BoitierD1Relais (Autodesk Fusion 360 design; units mm, degrees)
Autodesk Fusion 360 part; units mm, degrees
sketch "Esquisse1" plane through (0, 0, 0) normal (0, 0, 1) x (1, 0, 0) in component "Boitier"
  line L0 (-18, 13.5) -> (18, 13.5)
  line L1 (18, 13.5) -> (18, -13.5)
  line L2 (18, -13.5) -> (-18, -13.5)
  line L3 (-18, -13.5) -> (-18, 13.5)
  line L4 (-18, 13.5) -> (18, -13.5) construction
  line L5 (18, 13.5) -> (-18, -13.5) construction
  line L6 (19.5, -15) -> (-19.5, -15)
  line L7 (-19.5, -15) -> (-19.5, 15)
  line L8 (-19.5, 15) -> (19.5, 15)
  line L9 (19.5, 15) -> (19.5, -15)
  dimension "d4" = 36
  dimension "d5" = 27
  constraint horizontal L0
  constraint perpendicular L0 L1
  constraint parallel L0 L2
  constraint parallel L1 L3
  constraint coincident L4 origin
  constraint coincident L5 origin
  measures "d4" distance of L1.end L2.end
  measures "d5" distance of L0.end L1.end
extrude "Extrusion1" add sketch "Esquisse1" along normal blind 1.5 contours L0 L1 L2 L3 makes body 1 in component "Boitier"
extrude "Extrusion2" add sketch "Esquisse1" along normal blind 33 bodies 1 in component "Boitier"
fillet "Congé1" radius 3 3 edges at (19.5, -15, 16.5) (19.5, 15, 16.5) (-19.5, 15, 16.5) on bodies 1 in component "Boitier"
fillet "Congé2" radius 3 1 edges at (-19.5, -15, 16.5) on bodies 1 in component "Boitier"
fillet "Congé3" radius 1.5 1 edges at (18, 13.5, 17.25) on bodies 1 in component "Boitier"
fillet "Congé4" radius 1.5 1 edges at (18, -13.5, 17.25) on bodies 1 in component "Boitier"
fillet "Congé5" radius 1.5 1 edges at (-18, -13.5, 17.25) on bodies 1 in component "Boitier"
fillet "Congé6" radius 1.5 1 edges at (-18, 13.5, 17.25) on bodies 1 in component "Boitier"
fillet "Congé7" radius 0.1 8 edges at (-18.6213, -14.1213, 33) (0, -15, 33) (18.6213, -14.1213, 33) (19.5, 0, 33) (18.6213, 14.1213, 33) (0, 15, 33) (-18.6213, 14.1213, 33) (-19.5, 0, 33) on bodies 1 in component "Boitier"
sketch "Esquisse3" plane through (19.5, 0, 0) normal (1, 0, 0) x (0, 1, 0) in component "Boitier"
  line L0 (-12, 0) -> (12, 0)
  line L1 (6.5, 7.5) -> (-6.5, 7.5)
  line L2 (-6.5, 7.5) -> (-6.5, 1.5)
  line L3 (-6.5, 1.5) -> (6.5, 1.5)
  line L4 (6.5, 1.5) -> (6.5, 7.5)
  line L5 (6.5, 7.5) -> (-6.5, 1.5) construction
  line L6 (-6.5, 7.5) -> (6.5, 1.5) construction
  line L7 (15, 0) -> (-15, 0)
  line L8 (12, 32.9) -> (-12, 32.9)
  line L9 (-12, 32.9) -> (-12, 0)
  line L10 (12, 0) -> (12, 32.9)
  point P0 (0, 4.5)
  dimension "d31" = 13
  dimension "d32" = 6
  dimension "d34" = 1.5
  constraint horizontal L1
  constraint perpendicular L1 L2
  constraint parallel L1 L3
  constraint parallel L2 L4
  constraint coincident L5 P0
  constraint coincident L6 P0
  measures "d31" distance of L2.end L3.end
  measures "d32" distance of L1.end L2.end
  measures "d34" distance of L3 L7
extrude "Extrusion3" cut sketch "Esquisse3" against normal blind 1.7 contours L1 L2 L3 L4 bodies 1 in component "Boitier"
sketch "Esquisse4" plane through (-19.5, 0, 0) normal (-1, 0, 0) x (0, -1, 0) in component "Boitier"
  line L0 (-12, 0) -> (12, 0)
  circle A0 centre (0, 4.95) radius 2
  line L1 (12, 32.9) -> (-12, 32.9)
  line L2 (-12, 32.9) -> (-12, 0)
  line L3 (12, 0) -> (12, 32.9)
  dimension "d38" = 4
  dimension "d39" = 4.95
  measures "d38" diameter of A0
  measures "d39" distance of origin A0.centre
extrude "Extrusion4" cut sketch "Esquisse4" against normal blind 1.7 contours A0 bodies 1 in component "Boitier"
sketch "Esquisse1 (2)" plane through (0, 0, 0) normal (0, 0, 1) x (1, 0, 0) in component "Couvercle"
  line L0 (96, 38.5) -> (57, 38.5)
  line L1 (57, 38.5) -> (57, 8.5)
  line L2 (57, 8.5) -> (96, 8.5)
  line L3 (96, 8.5) -> (96, 38.5)
  line L4 (96, 38.5) -> (57, 8.5) construction
  line L5 (57, 38.5) -> (96, 8.5) construction
  point P0 (76.5, 23.5)
  dimension "d77" = 39
  dimension "d78" = 30
  constraint horizontal L0
  constraint perpendicular L0 L1
  constraint parallel L0 L2
  constraint parallel L1 L3
  constraint coincident L4 P0
  constraint coincident L5 P0
  measures "d77" distance of L1.end L2.end
  measures "d78" distance of L0.end L1.end
extrude "Extrusion1'" add sketch "Esquisse1 (2)" along normal blind 1.5 separate body makes body 2 in component "Couvercle"
sketch "Esquisse2" plane through (0, 0, 1.5) normal (0, 0, 1) x (-1, 0, 0) in component "Couvercle"
  line L0 (-96, -8.5) -> (-96, -38.5)
  line L1 (-96, -38.5) -> (-57, -38.5)
  line L2 (-57, -38.5) -> (-57, -8.5)
  line L3 (-57, -8.5) -> (-96, -8.5)
  line L4 (-58.55, -36.95) -> (-94.45, -36.95)
  line L5 (-94.45, -36.95) -> (-94.45, -10.05)
  line L6 (-94.45, -10.05) -> (-58.55, -10.05)
  line L7 (-58.55, -10.05) -> (-58.55, -36.95)
  dimension "d81" = 35.9
  dimension "d82" = 26.9
  dimension "d83" = 1.55
  dimension "d84" = 1.55
  constraint horizontal L4
  constraint vertical L5
  constraint horizontal L6
  constraint vertical L7
  measures "d81" distance of L4.start L4.end
  measures "d82" distance of L4.start L6.end
  measures "d83" distance of L2 L7
  measures "d84" distance of L1 L4
extrude "Extrusion2'" add sketch "Esquisse2" along normal blind 2.25 contours L4 L5 L6 L7 bodies 2 in component "Couvercle"
sketch "Esquisse3 (2)" plane through (0, 0, 3.75) normal (0, 0, 1) x (-1, 0, 0) in component "Couvercle"
  line L0 (-58.55, -10.05) -> (-94.45, -10.05)
  line L1 (-94.45, -10.05) -> (-94.45, -36.95)
  line L2 (-94.45, -36.95) -> (-58.55, -36.95)
  line L3 (-58.55, -36.95) -> (-58.55, -10.05)
  line L4 (-60.05, -35.45) -> (-93.05, -35.45)
  line L5 (-93.05, -35.45) -> (-93.05, -11.45)
  line L6 (-93.05, -11.45) -> (-60.05, -11.45)
  line L7 (-60.05, -11.45) -> (-60.05, -35.45)
  dimension "d87" = 33
  dimension "d88" = 24
  dimension "d89" = 1.5
  dimension "d90" = 1.5
  constraint horizontal L4
  constraint vertical L5
  constraint horizontal L6
  constraint vertical L7
  measures "d87" distance of L4.start L4.end
  measures "d88" distance of L4.start L6.end
  measures "d89" distance of L3 L7
  measures "d90" distance of L2 L4
extrude "Extrusion3'" cut sketch "Esquisse3 (2)" against normal blind 2.25 contours L4 L5 L6 L7 bodies 2 in component "Couvercle"
fillet "Congé1'" radius 1.5 1 edges at (94.45, 10.05, 2.625) on bodies 2 in component "Couvercle"
fillet "Congé2'" radius 1.5 2 edges at (94.45, 36.95, 2.625) (58.55, 10.05, 2.625) on bodies 2 in component "Couvercle"
fillet "Congé3'" radius 1.5 1 edges at (58.55, 36.95, 2.625) on bodies 2 in component "Couvercle"
fillet "Congé4'" radius 3 3 edges at (57, 38.5, 0.75) (96, 38.5, 0.75) (57, 8.5, 0.75) on bodies 2 in component "Couvercle"
fillet "Congé5'" radius 3 1 edges at (96, 8.5, 0.75) on bodies 2 in component "Couvercle"
fillet "Congé6'" radius 1.5 8 edges at (76.5, 38.5, 0) (57.8787, 37.6213, 0) (57, 23.5, 0) (57.8787, 9.3787, 0) (76.5, 8.5, 0) (95.1213, 9.3787, 0) (96, 23.5, 0) (95.1213, 37.6213, 0) on bodies 2 in component "Couvercle"
fillet "Congé8" radius 3 8 edges at (-18.6213, -14.1213, 0) (0, -15, 0) (18.6213, -14.1213, 0) (19.5, 0, 0) (18.6213, 14.1213, 0) (0, 15, 0) (-18.6213, 14.1213, 0) (-19.5, 0, 0) on bodies 1 in component "Boitier"
component "Boitier" placed x (1, 0, 0) y (0, 1, 0) z (0, 0, 1) at (0, 0, 0)
component "Couvercle" placed x (1, 0, 0) y (0, 1, 0) z (0, 0, 1) at (0, 0, 0)
equation "longueur_boitier = 36 mm"
equation "largeur_boitier = 27 mm"
equation "epaisseur = 1.5 mm"
equation "d4 = longueur_boitier"
equation "d5 = largeur_boitier"
equation "d6 = -epaisseur"
equation "d7 = epaisseur"
equation "hauteur_boite = 33 mm"
equation "d10 = hauteur_boite"
equation "rayon_ext = 3 mm"
equation "rayon_int = 1.5 mm"
equation "rayon_sur = 0.1 mm"
equation "d16 = rayon_ext"
equation "d18 = rayon_ext"
equation "d20 = rayon_int"
equation "d22 = rayon_int"
equation "d24 = rayon_int"
equation "d26 = rayon_int"
equation "d28 = rayon_sur"
equation "longueur_usb = 13 mm"
equation "hauteur_usb = 6 mm"
equation "d31 = longueur_usb"
equation "d32 = hauteur_usb"
equation "jeu = 0.2 mm"
equation "d34 = epaisseur"
equation "d35 = -epaisseur - jeu"
equation "diametre_cables = 4 mm"
equation "d38 = diametre_cables"
equation "d39 = 1.5 * ( hauteur_boite / 10 )"
equation "d40 = -epaisseur - jeu"
equation "d77 = longueur_boitier + epaisseur + epaisseur"
equation "d78 = largeur_boitier + epaisseur + epaisseur"
equation "d79 = epaisseur"
equation "d81 = longueur_boitier - jeu / 2"
equation "d82 = largeur_boitier - jeu / 2"
equation "d83 = epaisseur + jeu / 4"
equation "d84 = epaisseur + jeu / 4"
equation "d85 = epaisseur + epaisseur / 2"
equation "d87 = longueur_boitier - epaisseur - epaisseur"
equation "d88 = largeur_boitier - epaisseur - epaisseur"
equation "d89 = epaisseur"
equation "d90 = epaisseur"
equation "d91 = -epaisseur - epaisseur / 2"
equation "d94 = rayon_int"
equation "d96 = rayon_int"
equation "d98 = rayon_int"
equation "d100 = rayon_ext"
equation "d102 = rayon_ext"
equation "d104 = rayon_int"
equation "d106 = rayon_ext"
